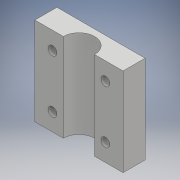
# Autodesk Inventor part: push_wall
Saved by Autodesk Inventor 2017 (Build 210142000, 142)
## iProperties
Part Number: push_wall
Material: Типовые
Document SubType Name: Modeling
Designer: Tolya
Density: 1 g/cm^3
Appearance: По умолчанию
Author: Tolya
## iProperties of the stored document push_wall_3DПЕЧАТЬ.ipt
Part Number: push_wall_3DПЕЧАТЬ
Material: Типовые
Document SubType Name: Modeling
Designer: Tolya
Density: 1 g/cm^3
Appearance: По умолчанию
Author: Tolya
Autodesk Inventor part; units mm, degrees
ref_plane "YZ Plane" through (0, 0, 0) normal (1, 0, 0) x (0, 1, 0)
ref_plane "XZ Plane" through (0, 0, 0) normal (0, 1, 0) x (-1, 0, 0)
ref_plane "XY Plane" through (0, 0, 0) normal (0, 0, 1) x (1, 0, 0)
sketch "Эскиз1" plane through (0, 0, 0) normal (0, 0, 1) x (1, 0, 0)
  line L0 (20, 0) -> (20, 5)
  line L1 (20, 5) -> (0, 5)
  line L2 (0, 5) -> (0, 0)
  arc A0 (13.55, 0) -> (6.45, 0) centre (10, 0) ccw
  line L3 (0, 0) -> (6.45, 0)
  line L4 (13.55, 0) -> (20, 0)
  dimension "d0" = 20
  dimension "d1" = 5
  dimension "d2" = 7.1
  constraints: 10 end point, 3 parallel, 2 horizontal, 2 perpendicular, 2 point on circle, 1 centre point
  measures "d0" distance of L1.end L0.end
  measures "d1" distance of L0.end L0.start
  measures "d2" diameter of A0
extrude "Выдавливание1" add sketch "Эскиз1" along normal blind 20
sketch "Эскиз2" plane through (0, 5, 0) normal (0, 1, 0) x (1, 0, 0)
  circle A0 centre (4, -4) radius 1
  circle A1 centre (4, -16) radius 1
  line L0 (13.55, -20) -> (6.45, -20) projected
  line L1 (6.45, 0) -> (13.55, 0) projected
  circle A2 centre (16, -4) radius 1
  circle A3 centre (16, -16) radius 1
  point P0 (0, 0)
  dimension "d5" = 2
  constraints: 4 centre point
  measures "d5" diameter of A0
extrude "Выдавливание2" cut sketch "Эскиз2" against normal blind 30
